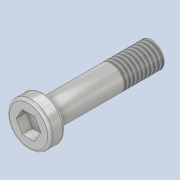
# Autodesk Inventor part: ScrewM5x40_Machined
Saved by Autodesk Inventor 2020.4 (Build 244396000, 396)
## iProperties
Created: 2019-04-17
Part Number: ScrewM5x40_Machined
Material: Aluminum 6061-AHC
Document SubType Name: Modeling
Designer: victo
Density: 2.7 g/cm^3
Appearance: Aluminum - Dark
Mass: 2.09572 g
Surface Area: 7.4105 cm^2
Volume: 0.776191 cm^3
Author: victo
Autodesk Inventor part; units mm, degrees
ref_plane "YZ Plane" through (0, 0, 0) normal (1, 0, 0) x (0, 1, 0)
ref_plane "XZ Plane" through (0, 0, 0) normal (0, 1, 0) x (-1, 0, 0)
sketch "Sketch1" plane through (0, 0, 0) normal (0, 0, 1) x (1, 0, 0)
  circle A0 centre (0, 0) radius 4.225
  dimension "d0" = 8.45
  constraints: 1 centre point, 1 coincident
  measures "d0" diameter of A0
extrude "Extrusion1" add sketch "Sketch1" against normal blind 3
sketch "Sketch2" plane through (0, 0, -3) normal (0, 0, -1) x (-1, 0, 0)
  circle A0 centre (0, 0) radius 2.475
  dimension "d3" = 4.95
  constraints: 1 centre point, 1 coincident
  measures "d3" diameter of A0
extrude "Extrusion2" add sketch "Sketch2" along normal blind 40
thread "Thread1" size "M5x0.8" class "6g" standard "ANSI Metric M Profile" length 27
sketch "Sketch3" plane through (0, 0, 0) normal (0, 0, 1) x (1, 0, 0)
  line L0 (-1.2124, -2.1) -> (-2.4249, 0)
  line L1 (-2.4249, 0) -> (-1.2124, 2.1)
  line L2 (-1.2124, 2.1) -> (1.2124, 2.1)
  line L3 (1.2124, 2.1) -> (2.4249, 0)
  line L4 (2.4249, 0) -> (1.2124, -2.1)
  line L5 (1.2124, -2.1) -> (-1.2124, -2.1)
  line L6 (-4.5, -0.75) -> (4.5, -0.75)
  line L7 (4.5, -0.75) -> (4.5, 0.75)
  line L8 (4.5, 0.75) -> (-4.5, 0.75)
  line L9 (-4.5, 0.75) -> (-4.5, -0.75)
  line L10 (-4.5, -0.75) -> (4.5, 0.75) construction
  line L11 (4.5, -0.75) -> (-4.5, 0.75) construction
  point P0 (0, 0)
  point P1 (0, 0)
  dimension "d8" = 2.1
  dimension "d13" = 4.2
  dimension "d18" = 9
  dimension "d19" = 1.5
  constraints: 24 end point, 2 midpoint, 2 parallel, 1 coincident, 1 horizontal, 1 perpendicular, 13 other
  measures "d8" distance from line of point (0, 0) L5
  measures "d13" vertical distance of L4.end L1.end
  measures "d18" distance of L8.end L7.end
  measures "d19" distance of L7.end L6.end
extrude "Extrusion3" cut sketch "Sketch3" against normal blind 2 contours L0 L6 L4 L5 | L0 L1 L8 L3 L4 L6 | L1 L2 L3 L8
fillet "Fillet1" radius 0.5 2 edges at (-4.225, 0, 0) (-4.225, 0, -3)
ref_plane "Work Plane1" through (0, 0, -18.5) normal (0, 0, -1) x (-1, 0, 0)
sketch "Sketch4" plane through (0, 0, -43) normal (0, 0, -1) x (-1, 0, 0)
  circle A0 centre (0, 0) radius 2.475 projected
extrude "Extrusion4" cut sketch "Sketch4" against normal blind 19
body "Solid1"
